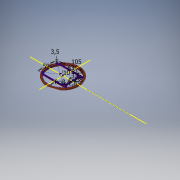
# Autodesk Inventor part: ODroid Xu4 Holder
Saved by Autodesk Inventor 2018 (Build 220112000, 112)
## iProperties
Part Number: ODroid Xu4 Holder
Material: Kupfer, Guss
Document SubType Name: Modeling
Designer: Jochen Alt
Mass: 179.761 g
Surface Area: 193.281 cm^2
Volume: 20.1075 cm^3
Density: 8.94 g/cm^3
Appearance: Kupfer - satiniert
Author: Jochen Alt
Autodesk Inventor part; units mm, degrees
ref_plane "YZ Plane" through (0, 0, 0) normal (1, 0, 0) x (0, 1, 0)
ref_plane "XZ Plane" through (0, 0, 0) normal (0, 1, 0) x (-1, 0, 0)
sketch "Skizze1" plane through (0, 0, 0) normal (0, 0, 1) x (1, 0, 0)
  circle A0 centre (0, 0) radius 59.3
  circle A1 centre (0, 0) radius 52.5
  circle A2 centre (0, 0) radius 53.6 construction
  line L0 (-83.17, 0) -> (83.92, 0) construction
  line L1 (35.006, -44.9842) -> (-1.8793, -56.969)
  line L2 (-54.7615, 15.817) -> (-31.9651, 47.1935)
  line L3 (-1.8793, 56.969) -> (35.006, 44.9842)
  line L4 (-31.9651, -47.1935) -> (-54.7615, -15.817)
  arc A3 (-31.9651, -47.1935) -> (-1.8793, -56.969) centre (0, 0) ccw
  arc A4 (-54.7615, 15.817) -> (-54.7615, -15.817) centre (0, 0) ccw
  arc A5 (35.006, -44.9842) -> (35.006, 44.9842) centre (0, 0) ccw
  arc A6 (-1.8793, 56.969) -> (-31.9651, 47.1935) centre (0, 0) ccw
  circle A7 centre (0, 0) radius 46.4646
  line L5 (16.5633, -50.9766) -> (0, 0) construction
  line L6 (0, 0) -> (-43.3633, -31.5053) construction
  line L7 (0, 0) -> (16.5633, 50.9766) construction
  line L8 (0, 0) -> (-43.3633, 31.5053) construction
  point P0 (60.05, 0)
  dimension "d7" = 118.6
  dimension "d100" = 105
  dimension "d108" = 107.2
  dimension "d110" = 57
  dimension "d115" = 6.0354
  dimension "d139" = 72
  dimension "d140" = 72
  dimension "d141" = 72
  dimension "d142" = 72
  constraints: 16 end point, 8 centre point, 8 point on circle, 6 coincident, 4 midpoint, 4 perpendicular, 3 concentric, 3 tangent, 2 other
  measures "d7" diameter of A0
  measures "d100" diameter of A1
  measures "d108" diameter of A2
  measures "d110" radius of A5
  measures "d115" radial gap between concentric circles of A7 A1
  measures "d139" angle of L5 L0
  measures "d140" angle of L0 L7
  measures "d141" angle of L7 L8
  measures "d142" angle of L6 L5
extrude "Extrusion3" add sketch "Skizze1" against normal blind 5 contours L1 A3 L4 A4 L2 A6 L3 A5
extrude "Extrusion4" add sketch "Skizze1" along normal blind 1.5 contours A0 | L1 A3 L4 A4 L2 A6 L3 A5
sketch "ODroidskizze" plane through (0, 0, 1.5) normal (0, 0, 1) x (1, 0, 0)
  line L0 (-120.4305, 0) -> (303.1004, 0) projected
  line L1 (28, -29.5) -> (-48, -29.5) construction
  line L2 (-51.5, -26) -> (-51.5, 26) construction
  line L3 (-48, 29.5) -> (28, 29.5) construction
  line L4 (31.5, 26) -> (31.5, -26) construction
  line L5 (31.5, -29.5) -> (-51.5, 29.5) construction
  line L6 (-51.5, -29.5) -> (31.5, 29.5) construction
  arc A0 (-48, 29.5) -> (-51.5, 26) centre (-48, 26) ccw construction
  arc A1 (31.5, 26) -> (28, 29.5) centre (28, 26) ccw construction
  arc A2 (28, -29.5) -> (31.5, -26) centre (28, -26) ccw construction
  arc A3 (-51.5, -26) -> (-48, -29.5) centre (-48, -26) ccw construction
  line L7 (-41.2311, 32.5) -> (41.2311, 32.5)
  line L8 (-41.2311, -32.5) -> (41.2311, -32.5)
  line L9 (242.596, 0) -> (86.2994, 0) construction
  line L10 (34.5, 26) -> (34.5, -26)
  line L11 (43.4281, 29.5) -> (38, 29.5)
  circle A4 centre (28, 26) radius 1.4
  circle A5 centre (28, -26) radius 1.4
  line L12 (24.5, -26) -> (24.5, -29.5)
  line L13 (28, -22.5) -> (31.5, -22.5)
  line L14 (24.5, 26) -> (24.5, 29.5)
  line L15 (28, 22.5) -> (31.5, 22.5)
  arc A6 (24.5, 26) -> (28, 22.5) centre (28, 26) ccw
  line L16 (43.4281, -29.5) -> (38, -29.5)
  line L17 (24.5, -29.5) -> (-43.4281, -29.5)
  arc A7 (28, -22.5) -> (24.5, -26) centre (28, -26) ccw
  line L18 (31.5, -22.5) -> (31.5, 22.5)
  arc A8 (38, 29.5) -> (34.5, 26) centre (38, 26) ccw
  arc A9 (34.5, -26) -> (38, -29.5) centre (38, -26) ccw
  line L19 (24.5, 29.5) -> (-43.4281, 29.5)
  arc A10 (-43.4281, -29.5) -> (-41.2311, -32.5) centre (0, 0) ccw
  arc A11 (-41.2311, 32.5) -> (-43.4281, 29.5) centre (0, 0) ccw
  arc A12 (41.2311, -32.5) -> (43.4281, -29.5) centre (0, 0) ccw
  arc A13 (43.4281, 29.5) -> (41.2311, 32.5) centre (0, 0) ccw
  circle A14 centre (0, 0) radius 52.5 construction
  line L20 (0, -85.9607) -> (0, 100.664) projected
  point P0 (-10, 0)
  point P1 (-42.3561, 31.0195)
  point P2 (-42.3561, -31.0195)
  point P3 (42.3561, -31.0195)
  point P4 (42.3561, 31.0195)
  dimension "d164" = 83
  dimension "d165" = 59
  dimension "d166" = 3.5
  dimension "d167" = 3
  dimension "d168" = 3
  dimension "d169" = 2.8
  dimension "d170" = 2.8
  dimension "d173" = 3.5
  dimension "d175" = 3.5
  dimension "d176" = 3.5
  dimension "d178" = 10
  dimension "d179" = 105
  constraints: 38 end point, 32 point on circle, 15 centre point, 14 point on line, 14 tangent, 7 horizontal, 4 equal radius, 4 parallel, 3 coincident, 3 collinear, 3 vertical, 2 concentric, 2 midpoint, 2 perpendicular, 3 other
  measures "d164" distance of L5.end L6.end
  measures "d165" distance of L5.end L6.start
  measures "d166" radius of A0
  measures "d167" distance between parallel lines of L3 L7
  measures "d168" distance between parallel lines of L10 L4
  measures "d169" diameter of A4
  measures "d170" diameter of A5
  measures "d173" radius of A8
  measures "d175" radius of A6
  measures "d176" radius of A7
  measures "d178" distance of A10.centre point (-10, 0)
  measures "d179" diameter of A14
extrude "Extrusion5" add sketch "ODroidskizze" against normal blind 3.5 contours L18 L15 A6 L14 L19 L20 L7 A13 L11 A8 L10 L0 | L0 L10 A9 L16 A12 L8 L20 L17 L12 A7 L13 L18 | L20 L8 A10 L17 | L19 A11 L7 L20
ref_plane "Arbeitsebene1" through (0, 0, -1) normal (0, 0, 1) x (1, 0, 0)
sketch "Skizze8" plane through (0, 0, 1.5) normal (0, 0, 1) x (1, 0, 0)
  arc A0 (41.2311, 32.5) -> (-41.2311, 32.5) centre (0, 0) ccw construction
  arc A1 (41.2311, 32.5) -> (-41.2311, 32.5) centre (0, 0) ccw construction
  circle A2 centre (-17.9561, -49.3339) radius 2
  circle A3 centre (-17.9561, 49.3339) radius 2
  line L0 (-83.02, 0) -> (83.02, 0) construction
  line L1 (-17.9561, -49.3339) -> (0, 0) construction
  line L2 (0, 0) -> (-17.9561, 49.3339) construction
  point P0 (52.5, 0)
  point P1 (52.5, 0)
  point P2 (52.5, 0)
  point P3 (52.5, 0)
  dimension "d116" = 4
  dimension "d117" = 4
  dimension "d143" = 70
  dimension "d144" = 70
  constraints: 4 end point, 4 point on circle, 2 centre point
  measures "d116" diameter of A2
  measures "d117" diameter of A3
  measures "d143" angle of L0 L1
  measures "d144" angle of L0 L2
extrude "Lidar-Holder-Nose" cut sketch "Skizze8" against normal up to next
chamfer "Fase5" distance 0.5 angle 45 16 edges at (-43.3633, -31.5053, -5) (-57, 0, -5) (-17.614, -54.2102, -5) (-43.3633, 31.5053, -5) (-17.614, 54.2102, -5) (16.5633, 50.9766, -5) (57, 0, -5) (16.5633, -50.9766, -5) (-31.5719, -41.9459, 1.5) (15.3216, -50.2145, 1.5) (15.3216, 50.2145, 1.5) (-31.5719, 41.9459, 1.5) (-52.5, 0, 1.5) (52.5, 0, 1.5) (-18.6401, 51.2132, 1.5) (-18.6401, -51.2132, 1.5)
